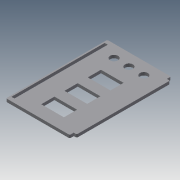
# Autodesk Inventor part: NewControlPanel
Saved by Autodesk Inventor 2014 (Build 180170000, 170)
## iProperties
Created: 2015-02-17
Part Number: NewControlPanel
Material: Generic
Document SubType Name: Modeling
Designer: Peele
Density: 1 g/cm^3
Appearance: Default
Author: Peele
Autodesk Inventor part; units mm, degrees
ref_plane "YZ Plane" through (0, 0, 0) normal (1, 0, 0) x (0, 1, 0)
ref_plane "XZ Plane" through (0, 0, 0) normal (0, 1, 0) x (-1, 0, 0)
ref_plane "XY Plane" through (0, 0, 0) normal (0, 0, 1) x (1, 0, 0)
sketch "Sketch1" plane through (0, 0, 0) normal (0, 0, 1) x (1, 0, 0)
  line L0 (0, 0) -> (128, 0)
  line L1 (128, 0) -> (128, 203.5927)
  line L2 (128, 203.5927) -> (0, 203.5927)
  line L3 (0, 203.5927) -> (0, 0)
  line L4 (0, 0) -> (-77.2375, 168.1052) construction
  line L5 (-77.2375, 168.1052) -> (0, 203.5927) construction
  line L6 (2.875, 195.5927) -> (9.125, 195.5927)
  line L7 (9.125, 195.5927) -> (9.125, 8)
  line L8 (9.125, 8) -> (2.875, 8)
  line L9 (2.875, 8) -> (2.875, 195.5927)
  dimension "d0" = 128
  dimension "d1" = 85
  dimension "d2" = 185
  dimension "d3" = 6.25
  dimension "d4" = 2.875
  dimension "d5" = 8
  dimension "d6" = 8
  constraints: 20 end point, 4 parallel, 3 perpendicular, 2 horizontal
  measures "d0" distance of L0.start L0.end
  measures "d1" distance from line of L2.end L4
  measures "d2" distance from line of L0.start L5
  measures "d3" distance of L6.start L6.end
  measures "d4" distance between parallel lines of L3 L9
  measures "d5" distance between parallel lines of L6 L2
  measures "d6" distance from line of L8.end L0
extrude "Extrusion1" add sketch "Sketch1" along normal blind 6
sketch "Sketch2" plane through (0, 0, 6) normal (0, 0, 1) x (1, 0, 0)
  line L0 (0, 0) -> (128, 0) projected
  line L1 (128, 0) -> (128, 203.5927) projected
  line L2 (128, 203.5927) -> (0, 203.5927) projected
  line L3 (128, 195.4927) -> (134, 195.4927)
  line L4 (134, 195.4927) -> (134, 8.1)
  line L5 (134, 8.1) -> (128, 8.1)
  line L6 (128, 8.1) -> (128, 195.4927)
  dimension "d9" = 8.1
  dimension "d10" = 8.1
  dimension "d11" = 6
  constraints: 8 end point, 2 parallel, 1 horizontal, 1 perpendicular, 1 point on line
  measures "d9" distance between parallel lines of L3 L2
  measures "d10" distance between parallel lines of L5 L0
  measures "d11" distance of L4.end L5.end
extrude "Extrusion2" add sketch "Sketch2" against normal blind 6
fillet "Fillet1" radius 2 6 edges at (134, 195.4927, 3) (128, 203.5927, 3) (0, 203.5927, 3) (128, 0, 3) (134, 8.1, 3) (0, 0, 3)
sketch "Sketch3" plane through (0, 0, 6) normal (0, 0, 1) x (1, 0, 0)
  line L0 (9.125, 195.5927) -> (9.125, 8) projected
  line L1 (2, 0) -> (126, 0) projected
  line L2 (128, 195.4927) -> (128, 201.5927) projected
  line L3 (126, 203.5927) -> (2, 203.5927) projected
  circle A0 centre (38.5625, 178.5927) radius 8
  circle A1 centre (68.5625, 178.5927) radius 8
  circle A2 centre (98.5625, 178.5927) radius 8
  line L4 (45.8125, 118.5618) -> (91.3125, 118.5618)
  line L5 (91.3125, 118.5618) -> (91.3125, 145.0618)
  line L6 (91.3125, 145.0618) -> (45.8125, 145.0618)
  line L7 (45.8125, 145.0618) -> (45.8125, 118.5618)
  line L8 (45.8125, 118.5618) -> (91.3125, 145.0618) construction
  line L9 (91.3125, 118.5618) -> (45.8125, 145.0618) construction
  line L10 (45.8125, 71.7809) -> (91.3125, 71.7809)
  line L11 (91.3125, 71.7809) -> (91.3125, 98.2809)
  line L12 (91.3125, 98.2809) -> (45.8125, 98.2809)
  line L13 (45.8125, 98.2809) -> (45.8125, 71.7809)
  line L14 (45.8125, 71.7809) -> (91.3125, 98.2809) construction
  line L15 (91.3125, 71.7809) -> (45.8125, 98.2809) construction
  line L16 (45.8125, 25) -> (91.3125, 25)
  line L17 (91.3125, 25) -> (91.3125, 51.5)
  line L18 (91.3125, 51.5) -> (45.8125, 51.5)
  line L19 (45.8125, 51.5) -> (45.8125, 25)
  line L20 (45.8125, 25) -> (91.3125, 51.5) construction
  line L21 (91.3125, 25) -> (45.8125, 51.5) construction
  line L22 (68.5625, 178.5927) -> (68.5625, 131.8118) construction
  line L23 (68.5625, 131.8118) -> (68.5625, 85.0309) construction
  line L24 (68.5625, 85.0309) -> (68.5625, 38.25) construction
  point P0 (0, 0)
  dimension "d15" = 16
  dimension "d16" = 26.5
  dimension "d17" = 45.5
  dimension "d18" = 118.875
  dimension "d19" = 59.4375
  dimension "d20" = 30
  dimension "d21" = 30
  dimension "d22" = 25
  dimension "d23" = 25
  constraints: 42 end point, 8 midpoint, 7 parallel, 6 equal length, 4 perpendicular, 3 centre point, 3 horizontal, 3 vertical alignment, 2 equal radius, 2 horizontal alignment
  measures "d15" diameter of A2
  measures "d16" distance of L4.end L5.end
  measures "d17" distance of L5.end L6.end
  measures "d18" distance between parallel lines of L0 L2
  measures "d19" distance from line of L22.start L0
  measures "d20" distance of A0.centre L22.start
  measures "d21" distance of L22.start A2.centre
  measures "d22" distance from line of A0.centre L3
  measures "d23" distance between parallel lines of L16 L1
extrude "Extrusion3" cut sketch "Sketch3" against normal blind 10
equation "\"d19\" = 0.5 * d18"
equation "\"d21\" = d20"
body "Solid1"
